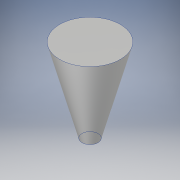
# Autodesk Inventor part: cone
Saved by Autodesk Inventor 2019 (Build 230136000, 136)
## iProperties
Created: 2019-08-21
Part Number: cone
Material: Aluminum 6061
Document SubType Name: Modeling
Designer: Dean
Density: 2.7 g/cm^3
Appearance: Aluminum - Flat
Author: Dean
Autodesk Inventor part; units mm, degrees
ref_plane "YZ Plane" through (0, 0, 0) normal (1, 0, 0) x (0, 1, 0)
ref_plane "XZ Plane" through (0, 0, 0) normal (0, 1, 0) x (-1, 0, 0)
ref_plane "XY Plane" through (0, 0, 0) normal (0, 0, 1) x (1, 0, 0)
sketch "Sketch1" plane through (0, 0, 0) normal (0, 0, 1) x (1, 0, 0)
  line L0 (0, 0.5) -> (0, 10)
  line L1 (0.9112, 0.5) -> (3.4567, 10)
  line L2 (0, 10) -> (3.4567, 10)
  line L3 (0, 0.5) -> (0.9112, 0.5)
  point P0 (0, 0)
  dimension "d0" = 10
  dimension "d1" = 15
  dimension "d3" = 9.5
  constraints: 8 end point, 1 horizontal, 1 perpendicular, 1 vertical
  measures "d0" distance of point (0, 0) L0.end
  measures "d1" angle of L0 L1
  measures "d3" distance between parallel lines of L3 L2
revolve "Revolution1" add sketch "Sketch1" angle 360 about axis through (0, 0.5, 0) along (0, 1, 0)
body "Solid1"
